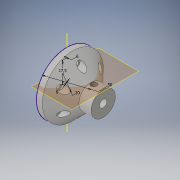
# Autodesk Inventor part: BT003_trajan20_21
Saved by Autodesk Inventor 2022.2 (Build 262287000, 287)
## iProperties
Company: HTBLA Kaindorf
RuleStatus: InUse
Created: 2022-08-01
Part Number: BT003_trajan20_21
Project: Zeichenmaschine_v2
Material: Generisch
Description: zwischenteil platte gm
Document SubType Name: Modeling
Designer: trajan20
Density: 1 g/cm^3
Appearance: Vorgabe
Mass: 26.4432 g
Surface Area: 72.75 cm^2
Volume: 26.4432 cm^3
AfterDocNew0: iProperties-Editor_aufrufen
Author: jan
Keywords: 2021
Autodesk Inventor part; units mm, degrees
note: some values were not read from the file. Chosen so that the rebuilt part matches the saved one: direction of "Bohrung1".
ref_plane "YZ Plane" through (0, 0, 0) normal (1, 0, 0) x (0, 1, 0)
ref_plane "XZ Plane" through (0, 0, 0) normal (0, 1, 0) x (-1, 0, 0)
sketch "Skizze3" plane through (0, 0, 0) normal (0, 1, 0) x (-1, 0, 0)
  circle A0 centre (0, 0) radius 25
  line L0 (0, -35) -> (0, 35) projected
  circle A1 centre (0, 0) radius 10
  circle A2 centre (0, 0) radius 3
  circle A3 centre (0, 17.5) radius 3
  dimension "d6" = 50
  dimension "d7" = 17.5
  dimension "d8" = 20
  dimension "d16" = 6
  dimension "d41" = 6
  constraints: 4 centre point, 4 coincident, 1 point on line
  measures "d6" diameter of A0
  measures "d7" distance of point (0, 0) point (0, 17.5)
  measures "d8" diameter of A1
  measures "d16" diameter of A2
  measures "d41" diameter of A3
extrude "Extrusion3" add sketch "Skizze3" along normal blind 30 contours A1 L0 A2 | L0 A2 A1 | A2 L0 | L0 A2
extrude "Extrusion4" add sketch "Skizze3" along normal blind 20 contours A0 L0 A1 A3 | L0 A3 A1 A0 | A3 L0 | L0 A3
chamfer "Fase1" distance 15 angle 45 1 edges at (25, 20, 0)
extrude "Extrusion5" cut sketch "Skizze3" along normal through all contours A2 L0 | L0 A2
extrude "Extrusion6" add sketch "Skizze3" along normal blind 15 contours A2 L0 | L0 A2
ref_plane "Arbeitsebene1" through (0, 0, 10) normal (0, 0, 1) x (1, 0, 0)
sketch "Skizze4" plane through (0, 0, 10) normal (0, 0, 1) x (1, 0, 0)
  line L0 (10, 20) -> (-10, 20) projected
  line L1 (10, 20) -> (10, 30) projected
  point P0 (0, 0)
  point P1 (0, 22.5)
  dimension "d22" = 2.5
  dimension "d23" = 10
  measures "d22" distance from line of L0 point (0, 22.5)
  measures "d23" distance from line of point (0, 22.5) L1
hole "Bohrung1" at (0, 22.5, 10) direction (0, 0, -1) diameter 4.4587 end up to surface thread size "M5x0.5" class "6H" standard "ISO Metric profile"
chamfer "Fase2" distance 0.2 angle 45 2 edges at (-2.2294, 22.4965, 9.7483) (2.2185, 22.7196, 9.7508)
sketch "Skizze5" plane through (0, 0, 0) normal (0, -1, 0) x (1, 0, 0)
  point P0 (0, 0)
extrude "Extrusion7" cut sketch "Skizze3" along normal blind 20 contours A3 L0 | L0 A3
extrude "Extrusion8" add sketch "Skizze3" along normal blind 8 contours A3 L0 | L0 A3
hole "Bohrung2" at (0, 0, 17.5) direction (0, 1, 0) diameter 3.5 depth 15
pattern_circular "Runde Anordnung1" count 6 over 360 about axis through (0, 0, 0) along (0, 1, 0) of "Extrusion7", "Bohrung2", "Extrusion8"
hole "Bohrung3" at (0, 0, 0) direction (0, 1, 0) diameter 5 depth 4
